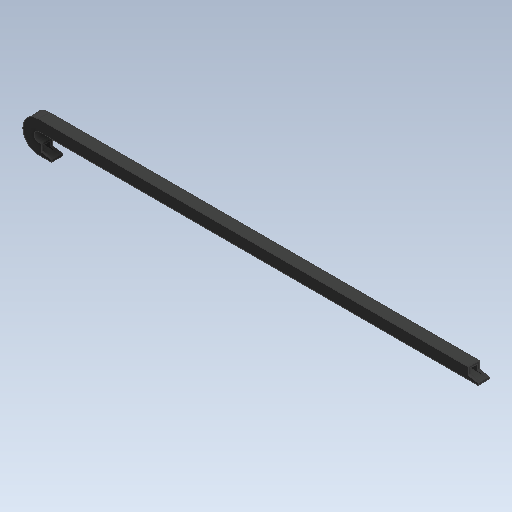
# Autodesk Inventor part: 0008-10-1025 Wire chain
Saved by Autodesk Inventor 2020 (Build 240168000, 168)
## iProperties
Created: 2021-03-13
Part Number: 0008-10-1025 Wire chain
Material: Generic
Document SubType Name: Modeling
Designer: Iulian Bors
Density: 1 g/cm^3
Appearance: Default
Description: Lant Portcablu
Mass: 33.8133 g
Surface Area: 340.239 cm^2
Volume: 33.8133 cm^3
Author: Iulian Bors
Subject: 1025
Autodesk Inventor part; units mm, degrees
ref_plane "YZ Plane" through (0, 0, 0) normal (1, 0, 0) x (0, 1, 0)
ref_plane "XZ Plane" through (0, 0, 0) normal (0, 1, 0) x (-1, 0, 0)
sketch "Sketch1" plane through (0, 0, 0) normal (0, 0, 1) x (1, 0, 0)
  line L0 (219, 20) -> (-219, 20)
  line L1 (-53.0332, 0) -> (53.0332, 0) construction
  arc A0 (-219, 20) -> (-219, 0) centre (-219, 10) ccw
  line L2 (-219, 0) -> (-205.9689, 0)
  point P0 (0, 0)
  point P1 (0, 20)
  point P2 (0, 0)
  dimension "d0" = 438
  dimension "d1" = 20
  constraints: 6 end point, 2 horizontal, 2 midpoint, 2 point on circle, 2 tangent, 1 centre point, 1 coincident, 1 parallel, 1 point on line, 1 vertical alignment
  measures "d0" distance of L0.start L0.end
  measures "d1" distance between parallel lines of L1 L0
ref_plane "Work Plane1" through (219, 20, 0) normal (-1, 0, 0) x (0, -1, 0)
sketch "Sketch2" plane through (219, 20, 0) normal (-1, 0, 0) x (0, -1, 0)
  line L0 (3.5, 3.5) -> (-3.5, 3.5)
  line L1 (-3.5, 3.5) -> (-3.5, -3.5)
  line L2 (-3.5, -3.5) -> (3.5, -3.5)
  line L3 (3.5, -3.5) -> (3.5, 3.5)
  line L4 (-5.5, 5.5) -> (5.5, 5.5)
  line L5 (5.5, 5.5) -> (5.5, -5.5)
  line L6 (5.5, -5.5) -> (-5.5, -5.5)
  line L7 (-5.5, -5.5) -> (-5.5, 5.5)
  point P0 (20, 0)
  point P1 (0, 3.5)
  point P2 (3.5, 0)
  point P3 (0, 0)
  point P4 (0, 0)
  point P5 (0, 0)
  dimension "d2" = 7
  dimension "d3" = 7
  dimension "d4" = 2
  constraints: 16 end point, 4 parallel, 2 midpoint, 2 perpendicular, 1 horizontal, 1 horizontal alignment, 1 vertical alignment, 3 other
  measures "d2" distance of L0.start L0.end
  measures "d3" distance of L0.end L1.end
  measures "d4" distance between parallel lines of L0 L4
sweep "Sweep1" add profiles "Sketch2" path "Sketch1"
sketch "Sketch3" plane through (219, 14.5, 5.5) normal (0, 0, 1) x (1, 0, 0)
  line L0 (-9.8481, 11) -> (0, 11)
  line L1 (0, 11) -> (0, 2)
  line L2 (-9.8481, 3.7365) -> (-9.8481, 11)
  line L3 (0, 11) -> (-438, 11) projected
  line L4 (0, 0) -> (0, 11) projected
  line L5 (0, 0) -> (-438, 0) projected
  line L6 (-9.8481, 3.7365) -> (0, 2)
  line L7 (-424.9689, -9) -> (-424.9689, -20) projected
  line L8 (-424.9689, -9) -> (-434.9689, -9)
  line L9 (-438, -9) -> (-424.9689, -9) projected
  line L10 (-434.9689, -9) -> (-434.9689, -6.6574)
  line L11 (-424.9689, -18) -> (-424.9689, -11) projected
  line L12 (-438, -20) -> (-424.9689, -20) projected
  line L13 (-434.9689, -9) -> (-434.9689, -16.2367)
  line L14 (-434.9689, -16.2367) -> (-424.9689, -18)
  point P0 (-219, -14.5)
  dimension "d7" = 10
  dimension "d9" = 100
  dimension "d10" = 2
  dimension "d13" = 10
  dimension "d18" = 100
  dimension "d19" = 2
  constraints: 16 end point, 2 collinear, 2 point on line, 2 vertical, 1 horizontal, 1 parallel, 1 perpendicular
  measures "d7" distance of L1.end L2.start
  measures "d9" angle of L2 L6
  measures "d10" distance from line of L5 L1.end
  measures "d13" distance of L7.start L8.end
  measures "d18" angle of L14 L13
  measures "d19" distance from line of L12 L14.end
extrude "Extrusion1" cut sketch "Sketch3" against normal through all
equation "\"d13\" = d7"
body "Solid1"
